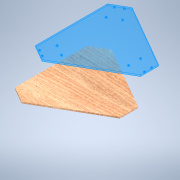
# Autodesk Inventor part: lap
Saved by Autodesk Inventor 2022 (Build 260153000, 153)
## iProperties
Created: 2021-10-06
Part Number: lap
Material: Wood (Birch)
Document SubType Name: Modeling
Designer: Varga Tamás
Density: 0.55 g/cm^3
Appearance: Birch - Natural Polished
Mass: 140.926 g
Surface Area: 1080.41 cm^2
Volume: 256.23 cm^3
Author: Varga Tamás
Autodesk Inventor part; units mm, degrees
ref_plane "YZ Plane" through (0, 0, 0) normal (1, 0, 0) x (0, 1, 0)
ref_plane "XZ Plane" through (0, 0, 0) normal (0, 1, 0) x (-1, 0, 0)
ref_plane "XY Plane" through (0, 0, 0) normal (0, 0, 1) x (1, 0, 0)
sketch "Sketch1" plane through (0, 0, 0) normal (0, 1, 0) x (-1, 0, 0)
  line L0 (-259.8076, 150) -> (-259.8076, 90)
  line L1 (-259.8076, 90) -> (-51.9615, -30)
  line L2 (-51.9615, -30) -> (0, 0)
  line L3 (0, 0) -> (0, 240)
  line L4 (0, 240) -> (-51.9615, 270)
  line L5 (-51.9615, 270) -> (-259.8076, 150)
  dimension "d0" = 120
  dimension "d1" = 120
  dimension "d2" = 120
  dimension "d4" = 120
  dimension "d5" = 120
  dimension "d6" = 60
  dimension "d7" = 120
  dimension "d71" = 259.8076
  dimension "d72" = 300
  constraints: 13 end point, 2 equal length, 1 vertical
  measures "d0" angle of L4 L5
  measures "d1" angle of L3 L2
  measures "d2" angle of L1 L0
  measures "d4" angle of L1 L2
  measures "d5" angle of L3 L4
  measures "d6" distance of L0.start L0.end
  measures "d7" vertical distance of L4.end L0.start
  measures "d71" distance from line of L0.end L3
  measures "d72" distance of L1.end L4.end
extrude "Extrusion1" add sketch "Sketch1" along normal blind 5
sketch "Sketch2" plane through (0, 5, 0) normal (0, 1, 0) x (1, 0, 0)
  line L0 (254.8076, -108) -> (254.8076, -132)
  line L1 (259.8076, -150) -> (259.8076, -90) projected
  line L2 (259.8076, -90) -> (51.9615, 30) projected
  line L3 (51.9615, -270) -> (259.8076, -150) projected
  line L4 (209.8076, -108) -> (209.8076, -132)
  line L5 (209.8076, -108) -> (209.8076, -100)
  line L6 (209.8076, -144.7569) -> (209.8076, -140)
  point P0 (0, 0)
  dimension "d10" = 24
  dimension "d11" = 5
  dimension "d12" = 18
  dimension "d31" = 18.0885
  dimension "d32" = 18.0885
  dimension "d33" = 18
  dimension "d44" = 45
  dimension "d45" = 0
  dimension "d47" = 40.5885
  dimension "d51" = 8
  dimension "d52" = 8
  constraints: 8 end point, 6 coincident, 3 vertical, 2 parallel, 1 collinear
  measures "d10" distance of L0.start L0.end
  measures "d11" distance between parallel lines of L1 L0
  measures "d12" vertical distance of L1.end L0.start
  measures "d31" distance from line of L2 L0.start
  measures "d32" distance from line of L3 L0.end
  measures "d33" vertical distance of L1.start L0.end
  measures "d44" distance between parallel lines of L0 L4
  measures "d45" vertical distance of L0.start L4.start
  measures "d47" distance from line of L2 L4.start
  measures "d51" distance of L5.start L5.end
  measures "d52" distance of point (209.808, -132) L6.end
hole "Hole1" at (209.8076, 5, 100) at (209.8076, 5, 140) at (254.8076, 5, 108) at (254.8076, 5, 132) direction (0, -1, 0) diameter 2.8 end through all
sketch "Sketch3" plane through (0, 5, 0) normal (0, 1, 0) x (1, 0, 0)
  line L0 (18.088, 4.6696) -> (38.8735, 16.6701)
  line L1 (51.9615, 30) -> (0, 0) projected
  line L2 (0, 0) -> (0, -240) projected
  line L3 (259.8076, -90) -> (51.9615, 30) projected
  line L4 (51.413, -28.0517) -> (72.1985, -16.0512)
  line L5 (72.1985, -16.0512) -> (68.3015, -18.3011)
  line L6 (51.413, -28.0517) -> (33.66, -38.3014)
  dimension "d20" = 5
  dimension "d22" = 18.088
  dimension "d23" = 18.088
  dimension "d46" = 45
  dimension "d53" = 33.66
  dimension "d73" = 33.66
  constraints: 8 end point, 6 coincident, 3 parallel, 2 collinear
  measures "d20" distance from line of L1.end L0
  measures "d22" distance from line of L0.start L2
  measures "d23" distance from line of L3 L0.end
  measures "d46" distance between parallel lines of L4 L0
  measures "d53" distance from line of L3 L5.end
  measures "d73" distance from line of L2 point (33.66, -38.301)
hole "Hole2" at (68.3015, 5, 18.3011) at (33.66, 5, 38.3014) at (18.088, 5, -4.6696) at (38.8735, 5, -16.6701) direction (0, -1, 0) diameter 2.8 end through all
sketch "Sketch4" plane through (0, 5, 0) normal (0, 1, 0) x (1, 0, 0)
  line L0 (18.088, -244.6696) -> (38.8735, -256.6701)
  line L1 (0, -240) -> (51.9615, -270) projected
  line L2 (51.9615, -270) -> (259.8076, -150) projected
  line L3 (0, 0) -> (0, -240) projected
  line L4 (47.516, -209.6983) -> (68.3015, -221.6989)
  line L5 (68.3015, -221.6989) -> (68.3015, -221.6989)
  line L6 (25.866, -197.1987) -> (33.66, -201.6986)
  dimension "d34" = 5
  dimension "d35" = 18.088
  dimension "d36" = 18.088
  dimension "d49" = 45
  dimension "d74" = 33.66
  dimension "d75" = 33.66
  dimension "d76" = 33.66
  constraints: 8 end point, 5 coincident, 3 parallel, 2 collinear
  measures "d34" distance between parallel lines of L1 L0
  measures "d35" distance from line of L2 L0.end
  measures "d36" distance from line of L3 L0.start
  measures "d49" distance between parallel lines of L4 L0
  measures "d74" distance from line of L2 L5.start
  measures "d75" distance from line of L3 point (33.66, -201.699)
  measures "d76" distance from line of L2 point (68.302, -221.699)
hole "Hole3" at (68.3015, 5, 221.6989) at (33.66, 5, 201.6986) at (18.088, 5, 244.6696) at (38.8735, 5, 256.6701) direction (0, -1, 0) diameter 2.8 end through all
sketch "Sketch5" plane through (0, 0, 0) normal (0, -1, 0) x (1, 0, 0)
  circle A0 centre (18.088, 244.6696) radius 1.4 projected
  circle A1 centre (68.3015, 221.6989) radius 1.4 projected
  circle A2 centre (33.66, 201.6986) radius 1.4 projected
  circle A3 centre (38.8735, 256.6701) radius 1.4 projected
  circle A4 centre (18.088, -4.6696) radius 1.4 projected
  circle A5 centre (68.3015, 18.3011) radius 1.4 projected
  circle A6 centre (33.66, 38.3014) radius 1.4 projected
  circle A7 centre (38.8735, -16.6701) radius 1.4 projected
  circle A8 centre (254.8076, 108) radius 1.4 projected
  circle A9 centre (209.8076, 100) radius 1.4 projected
  circle A10 centre (209.8076, 140) radius 1.4 projected
  circle A11 centre (254.8076, 132) radius 1.4 projected
  line L0 (259.8076, 90) -> (51.9615, -30) projected
  line L1 (259.8076, 150) -> (259.8076, 90) projected
  line L2 (51.9615, 270) -> (259.8076, 150) projected
  line L3 (0, 240) -> (51.9615, 270) projected
  line L4 (0, 0) -> (0, 240) projected
  line L5 (51.9615, -30) -> (0, 0) projected
  circle A12 centre (254.8076, 108) radius 1.4 projected
  circle A13 centre (254.8076, 108) radius 3
  circle A14 centre (254.8076, 132) radius 1.4 projected
  circle A15 centre (254.8076, 132) radius 3
  circle A16 centre (209.8076, 100) radius 3
  circle A17 centre (209.8076, 140) radius 3
  circle A18 centre (68.3015, 221.6989) radius 1.4 projected
  circle A19 centre (68.3015, 221.6989) radius 3
  circle A20 centre (38.8735, 256.6701) radius 1.4 projected
  circle A21 centre (38.8735, 256.6701) radius 3
  circle A22 centre (18.088, 244.6696) radius 1.4 projected
  circle A23 centre (18.088, 244.6696) radius 3
  circle A24 centre (33.66, 201.6986) radius 3
  circle A25 centre (33.66, 38.3014) radius 1.4 projected
  circle A26 centre (33.66, 38.3014) radius 3
  circle A27 centre (68.3015, 18.3011) radius 1.4 projected
  circle A28 centre (68.3015, 18.3011) radius 3
  circle A29 centre (38.8735, -16.6701) radius 1.4 projected
  circle A30 centre (38.8735, -16.6701) radius 3
  circle A31 centre (18.088, -4.6696) radius 1.4 projected
  circle A32 centre (18.088, -4.6696) radius 3
  dimension "d57" = 6
  dimension "d58" = 6
  dimension "d59" = 6
  dimension "d60" = 6
  dimension "d61" = 6
  dimension "d62" = 6
  dimension "d63" = 6
  dimension "d64" = 6
  dimension "d65" = 6
  dimension "d66" = 6
  dimension "d67" = 6
  dimension "d68" = 6
  constraints: 13 coincident, 12 centre point
  measures "d57" diameter of A13
  measures "d58" diameter of A15
  measures "d59" diameter of A16
  measures "d60" diameter of A17
  measures "d61" diameter of A19
  measures "d62" diameter of A21
  measures "d63" diameter of A23
  measures "d64" diameter of A24
  measures "d65" diameter of A26
  measures "d66" diameter of A28
  measures "d67" diameter of A30
  measures "d68" diameter of A32
extrude "Extrusion2" cut sketch "Sketch5" against normal blind 2.3 contours A13 | A15 | A16 | A17 | A19 | A21 | A23 | A24 | A26 | A28 | A30 | A32
body "Solid1"
